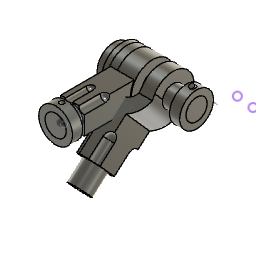
Knuckle Joint final_ (Autodesk Fusion 360 design; units mm, degrees)
Autodesk Fusion 360 part; units mm, degrees
sketch "Sketch1" plane through (0, 0, 0) normal (0, 1, 0) x (1, 0, 0) in component "eye"
  circle A0 centre (0, 0) radius 12.5
  dimension "d1" = 25
  constraint coincident A0.centre origin
  measures "d1" diameter of A0
extrude "Extrude1" add sketch "Sketch1" along normal blind 20 makes body 1 in component "eye"
sketch "Sketch2" plane through (0, 0, 0) normal (1, 0, 0) x (0, 1, 0) in component "eye"
sketch "Sketch3" plane through (0, 0, 0) normal (1, 0, 0) x (0, 1, 0) in component "eye"
  line L0 (20, 0) -> (100, 0)
  circle A0 centre (100, 0) radius 25
  circle A1 centre (100, 0) radius 12.5
  dimension "d4" = 80
  dimension "d5" = 50
  dimension "d6" = 25
  constraint coincident L0.end A0.centre
  constraint concentric A0 A1
  measures "d4" distance of L0.start L0.end
  measures "d5" diameter of A0
  measures "d6" diameter of A1
extrude "Extrude2" add sketch "Sketch3" along normal mid plane 30 separate body makes body 2 in component "eye"
sketch "Sketch4" plane through (0, 20, 0) normal (0, 1, 0) x (-1, 0, 0) in component "eye"
  circle A0 centre (0, 0) radius 12.5
sketch "Sketch1 (2)" plane through (0, 20, 0) normal (0, 1, 0) x (-1, 0, 0)
  line L0 (14, -14) -> (-14, -14)
  line L1 (-14, -14) -> (-14, 14)
  line L2 (-14, 14) -> (14, 14)
  line L3 (14, 14) -> (14, -14)
  line L4 (14, -14) -> (-14, 14) construction
  line L5 (-14, -14) -> (14, 14) construction
  dimension "d9" = 28
  dimension "d10" = 28
  constraint horizontal L0
  constraint perpendicular L0 L1
  constraint parallel L0 L2
  constraint parallel L1 L3
  constraint coincident L4 origin
  constraint coincident L5 origin
  measures "d9" distance of L0.start L0.end
  measures "d10" distance of L0.start L2.end
extrude "Extrude3" add sketch "Sketch1 (2)" along normal blind 60 bodies 1 2 in component "eye"
sketch "Sketch2 (2)" plane through (0, 0, 0) normal (0, 0, 1) x (1, 0, 0)
sketch "Sketch3 (2)" plane through (0, 0, 0) normal (0, 1, 0) x (1, 0, 0)
sketch "Sketch4 (2)" plane through (0, 0, 0) normal (0, 0, 1) x (1, 0, 0)
sketch "Sketch5" plane through (0, 0, 0) normal (0, 0, 1) x (1, 0, 0)
sketch "Sketch6" plane through (0, 0, 0) normal (0, 0, 1) x (1, 0, 0)
sketch "Sketch1 (3)" plane through (0, 0, 0) normal (0, 1, 0) x (1, 0, 0) in component "fork"
  arc A0 (3.8859, 308.1162) -> (3.8859, 278.1162) centre (3.8859, 293.1162) ccw
  arc A1 (3.8859, 323.1162) -> (3.8859, 263.1162) centre (3.8859, 293.1162) ccw
  line L0 (3.8859, 308.1162) -> (36.5811, 308.1162)
  line L1 (36.5811, 308.1162) -> (36.5811, 323.1162)
  line L2 (36.5811, 323.1162) -> (3.8859, 323.1162)
  line L3 (3.8859, 278.1162) -> (36.5811, 278.1162)
  line L4 (36.5811, 278.1162) -> (36.5811, 263.1162)
  line L5 (36.5811, 263.1162) -> (3.8859, 263.1162)
  line L6 (-22.6471, 307.1162) -> (-71.1141, 307.1162)
  line L7 (-71.1141, 307.1162) -> (-71.1141, 279.1162)
  line L8 (-71.1141, 279.1162) -> (-22.6471, 279.1162)
  dimension "d32" = 15
  dimension "d33" = 30
  dimension "d34" = 28
  dimension "d35" = 75
  constraint coincident A0.centre A1.centre
  constraint tangent A0 L0
  constraint horizontal L0
  constraint perpendicular L0 L1
  constraint tangent A1 L2
  constraint tangent A0 L3
  constraint parallel L2 L3
  constraint perpendicular L3 L4
  constraint tangent A1 L5
  constraint horizontal L6
  constraint perpendicular L6 L7
  constraint parallel L6 L8
  constraint coincident A1 L6.start
  constraint parallel L3 L5
  constraint parallel L0 L2
  constraint collinear L1 L4
  constraint coincident A1 L8.end
  constraint equal L6 L8
  measures "d32" radius of A0
  measures "d33" radius of A1
  measures "d34" distance of L6.end L7.end
  measures "d35" distance of A0.centre L7
extrude "Extrude1'" add sketch "Sketch1 (3)" along normal mid plane 56 separate body makes body 3 in component "fork"
sketch "Sketch2 (3)" plane through (0, 0, -263.1162) normal (0, 0, 1) x (-1, 0, 0) in component "fork"
  line L0 (-36.5811, 28) -> (-36.5811, -28)
  line L1 (-36.5811, -28) -> (-3.8859, -28)
  line L2 (-3.8859, -28) -> (-3.8859, 28)
  line L3 (-3.8859, 28) -> (-36.5811, 28)
  circle A0 centre (-11.5811, 0) radius 25
  circle A1 centre (-11.5811, 0) radius 12.5
  line L4 (1.9836, -21) -> (80, -21)
  line L5 (80, -21) -> (80, 21)
  line L6 (80, 21) -> (1.9836, 21)
  line L7 (1.9836, 21) -> (1.9836, -21)
  dimension "d38" = 50
  dimension "d39" = 25
  dimension "d40" = 42
  constraint concentric A0 A1
  constraint tangent L0 A0
  constraint horizontal L4
  constraint vertical L5
  constraint horizontal L6
  constraint vertical L7
  constraint coincident A0 L4.start
  constraint coincident A0 L6.end
  measures "d38" diameter of A0
  measures "d39" diameter of A1
  measures "d40" distance of L4.end L5.end
extrude "Extrude2'" cut sketch "Sketch2 (3)" against normal blind 80 contours L2 A0 A1 | L2 A0 A1 L7 | A0 L4 L5 L6 | A0 L7 keep common part bodies 3 in component "fork"
sketch "Sketch3 (3)" plane through (0, 0, 0) normal (0, 0, 1) x (1, 0, 0) in component "fork"
sketch "Sketch4 (3)" plane through (-71.1141, 0, 0) normal (-1, 0, 0) x (0, -1, 0) in component "fork"
  line L0 (21, -307.1162) -> (21, -279.1162)
  line L1 (21, -279.1162) -> (-21, -279.1162)
  line L2 (-21, -279.1162) -> (-21, -307.1162)
  line L3 (-21, -307.1162) -> (21, -307.1162)
  circle A0 centre (-0.0133, -293.1162) radius 12.5
  dimension "d45" = 25
  measures "d45" diameter of A0
extrude "Extrude3'" add sketch "Sketch4 (3)" along normal blind 25 contours A0 bodies 3 in component "fork"
sketch "Sketch5 (2)" plane through (0, 0, -279.1162) normal (0, 0, 1) x (-1, 0, 0) in component "fork"
  line L0 (71.1141, 21) -> (22.6471, 21)
  line L1 (22.6471, 21) -> (22.6471, -21)
  line L2 (22.6471, -21) -> (71.1141, -21)
  line L3 (71.1141, -21) -> (71.1141, 21)
  line L4 (71.1141, -12.4547) -> (48.3844, -12.4547)
  arc A0 (48.3844, -12.4547) -> (41.1141, -21) centre (48.3844, -19.82) ccw
  line L5 (71.1141, -21) -> (71.1141, -12.4547)
  dimension "d48" = 30
  dimension "d49" = 22.7298
  dimension "d50" = 7.3654
  constraint coincident L3 L4.start
  constraint perpendicular L3 L4
  constraint coincident L2 A0.end
  constraint tangent L4 A0
  constraint coincident L2.end L3.start
  measures "d48" horizontal distance of L4.start A0.end
  measures "d49" distance of L4.start L4.end
  measures "d50" radius of A0
revolve "Revolve1" cut sketch "Sketch5 (2)" angle 360 about axis through (-22.6471, 21, -279.1162) along (-1, 0, 0) contours L2 L3 L4 A0 L5 bodies 3 in component "fork"
sketch "Sketch6 (2)" plane through (0, 0, 0) normal (0, 0, 1) x (1, 0, 0) in component "fork"
sketch "Sketch7" plane through (0, 0, 0) normal (0, 0, 1) x (1, 0, 0) in component "fork"
sketch "Sketch7 (2)" plane through (0, 0, -79.4292) normal (0, 0, 1) x (-1, 0, 0)
  line L0 (128.0731, -132.4529) -> (150.8028, -132.4529)
  line L1 (150.8028, -132.4529) -> (150.8028, -98.9982)
  line L2 (150.8028, -98.9982) -> (102.3358, -98.9982)
  line L3 (102.3358, -98.9982) -> (102.3358, -140.9982)
  line L4 (102.3358, -140.9982) -> (120.8028, -140.9982)
  arc A0 (128.0731, -132.4529) -> (120.8028, -140.9982) centre (128.0731, -139.8183) ccw
  line L5 (150.8028, -107.545) -> (150.8028, -98.9982)
  line L6 (150.8028, -107.545) -> (128.0728, -107.545)
  arc A1 (120.8028, -98.9982) -> (128.0728, -107.545) centre (128.0728, -100.1796) ccw
  line L7 (150.8028, -98.9982) -> (120.8028, -98.9982)
  dimension "d52" = 22.73
  dimension "d53" = 30
  dimension "d54" = 7.3654
  constraint coincident L1 L5.start
  constraint coincident L1.end L2.start
  constraint perpendicular L2 L5
  constraint perpendicular L1 L6
  constraint coincident L2 A1.start
  constraint tangent L6 A1
  constraint equal A0 A1
  measures "d52" distance of L5.start L6.end
  measures "d53" horizontal distance of L5.start A1.start
  measures "d54" radius of A0
sketch "Sketch8" plane through (0, 0, -79.4292) normal (0, 0, 1) x (1, 0, 0)
sketch "Sketch9" plane through (0, 140.9982, 0) normal (0, 1, 0) x (-1, 0, 0)
  line L0 (150.8028, -87.9745) -> (128.0731, -87.9745)
  arc A0 (120.8028, -79.4292) -> (128.0731, -87.9745) centre (128.0731, -80.6092) ccw
  line L1 (120.8028, -79.4292) -> (102.3358, -79.4292)
  arc A1 (102.3358, -79.4292) -> (81.6723, -64.009) centre (75.8028, -93.4292) ccw
  line L2 (81.6723, -64.009) -> (81.6723, -79.6252)
  arc A2 (81.6723, -107.2332) -> (81.6723, -79.6252) centre (75.8028, -93.4292) ccw
  line L3 (81.6723, -107.2332) -> (81.6723, -122.8494)
  arc A3 (81.6723, -122.8494) -> (102.3358, -107.4292) centre (75.8028, -93.4292) ccw
  line L4 (102.3358, -107.4292) -> (150.8028, -107.4292)
  line L5 (150.8028, -107.4292) -> (150.8028, -87.9745)
  line L6 (150.8028, -107.4292) -> (150.8028, -98.8851)
  line L7 (150.8028, -98.8851) -> (128.0728, -98.8851)
  arc A4 (128.0728, -98.8851) -> (120.8028, -107.4292) centre (128.0728, -106.2501) ccw
  line L8 (120.8028, -107.4292) -> (150.8028, -107.4292)
  dimension "d58" = 30
  dimension "d59" = 7.365
  dimension "d60" = 22.73
  constraint coincident L4.end L5.start
  constraint coincident L5 L6.end
  constraint perpendicular L4 L6
  constraint perpendicular L5 L7
  constraint coincident L4 A4.end
  constraint tangent L7 A4
  measures "d58" horizontal distance of L6.end A4.end
  measures "d59" radius of A4
  measures "d60" distance of L6.end L7.end
sketch "Sketch10" plane through (0, 98.9982, 0) normal (0, -1, 0) x (1, 0, 0)
  arc A0 (-81.6723, -64.009) -> (-102.3358, -79.4292) centre (-75.8028, -93.4292) ccw
  line L0 (-102.3358, -79.4292) -> (-150.8028, -79.4292)
  line L1 (-150.8028, -79.4292) -> (-150.8028, -107.4292)
  line L2 (-150.8028, -107.4292) -> (-102.3358, -107.4292)
  arc A1 (-102.3358, -107.4292) -> (-81.6723, -122.8494) centre (-75.8028, -93.4292) ccw
  line L3 (-81.6723, -122.8494) -> (-81.6723, -107.2332)
  arc A2 (-81.6723, -79.6252) -> (-81.6723, -107.2332) centre (-75.8028, -93.4292) ccw
  line L4 (-81.6723, -79.6252) -> (-81.6723, -64.009)
revolve "Revolve2" cut sketch "Sketch7 (2)" angle 360 about axis through (-22.6471, -21, -279.1162) along (-1, 0, 0) contours L1 L2 L5 L6 A1 L7 sketch seen with x (1, 0, 0) y (0, 1, 0) z (0, 0, 1) at (79.6887, -119.9982, -199.687) bodies 3 in component "fork"
revolve "Revolve3" cut sketch "Sketch9" angle 360 about axis through (-22.6471, 21, -307.1162) along (-1, 0, 0) contours L4 L5 L6 L7 A4 L8 sketch seen with x (1, 0, 0) y (0, 1, 0) z (0, 0, 1) at (79.6887, -119.9982, -199.687) bodies 3 in component "fork"
sketch "Sketch11" plane through (0, 0, -107.4292) normal (0, 0, -1) x (1, 0, 0)
  arc A0 (-120.8028, -140.9982) -> (-128.0728, -132.4541) centre (-128.0728, -139.8191) ccw
  line L0 (-120.8028, -140.9982) -> (-102.3358, -140.9982)
  line L1 (-102.3358, -140.9982) -> (-102.3358, -98.9982)
  line L2 (-102.3358, -98.9982) -> (-150.8028, -98.9982)
  line L3 (-150.8028, -98.9982) -> (-150.8028, -132.4541)
  line L4 (-150.8028, -132.4541) -> (-128.0728, -132.4541)
  line L5 (-150.8028, -98.9982) -> (-150.8028, -107.0956)
  line L6 (-150.8028, -107.0956) -> (-128.0728, -107.0956)
  arc A1 (-128.0728, -107.0956) -> (-120.8028, -98.5514) centre (-128.0728, -99.7306) ccw
  line L7 (-120.8028, -98.5514) -> (-150.8028, -98.9982)
  dimension "d64" = 30
  dimension "d65" = 22.73
  dimension "d66" = 7.365
  constraint coincident L2.end L3.start
  constraint coincident L3 L5.end
  constraint perpendicular L2 L5
  constraint perpendicular L3 L6
  constraint tangent L6 A1
  constraint equal L4 L6
  constraint equal A0 A1
  measures "d64" horizontal distance of L5.end A1.end
  measures "d65" distance of L5.end L6.end
  measures "d66" radius of A1
revolve "Revolve4" cut sketch "Sketch11" angle 360 about axis through (-22.6471, -21, -307.1162) along (-1, 0, 0) contours L2 L3 L5 L6 A1 sketch seen with x (1, 0, 0) y (0, 1, 0) z (0, 0, 1) at (79.6887, -119.9982, -199.687) bodies 3 in component "fork"
sketch "Sketch1 (4)" plane through (0, 0, 0) normal (0, 1, 0) x (1, 0, 0) in component "pin"
  circle A0 centre (0, 0) radius 20
  dimension "d68" = 40
  constraint coincident A0.centre origin
  measures "d68" diameter of A0
extrude "Extrude1''" add sketch "Sketch1 (4)" along normal blind 12 separate body makes body 4 in component "pin"
sketch "Sketch2 (4)" plane through (0, 0, 0) normal (0, -1, 0) x (1, 0, 0) in component "pin"
  circle A0 centre (0, 0) radius 20
  circle A1 centre (0, 0) radius 12.5
  dimension "d71" = 25
  constraint coincident A0.centre A1.centre
  measures "d71" diameter of A1
extrude "Extrude2''" add sketch "Sketch2 (4)" along normal blind 86 contours A1 bodies 4 in component "pin"
sketch "Sketch3 (4)" plane through (0, 0, 0) normal (0, 0, 1) x (1, 0, 0) in component "pin"
sketch "Sketch4 (4)" plane through (0, 0, 0) normal (0, 1, 0) x (1, 0, 0) in component "pin"
sketch "Sketch1 (5)" plane through (0, 0, 0) normal (1, 0, 0) x (0, 0, -1) in component "collar"
  circle A0 centre (0, 0) radius 20
  circle A1 centre (0, 0) radius 12.5
  dimension "d74" = 40
  dimension "d75" = 25
  constraint coincident A0.centre A1.centre
  measures "d74" diameter of A0
  measures "d75" diameter of A1
extrude "Extrude1'''" add sketch "Sketch1 (5)" along normal blind 12 separate body makes body 5 in component "collar"
sketch "Sketch2 (5)" plane through (0, 0, 0) normal (0, 1, 0) x (1, 0, 0) in component "collar"
sketch "Sketch3 (5)" plane through (0, 0, 0) normal (0, 1, 0) x (1, 0, 0) in component "collar"
sketch "Sketch12" plane through (0, 0, 0) normal (1, 0, 0) x (0, 0, -1)
  circle A0 centre (0, -62.6322) radius 2
  line L0 (-10.0222, -74.6322) -> (14.9778, -74.6322)
  dimension "d80" = 4
  dimension "d81" = 12
  constraint vertical origin A0.centre
  measures "d80" diameter of A0
  measures "d81" distance of A0.centre L0
extrude "Extrude3''" cut sketch "Sketch12" along normal blind 28 sketch seen with x (1, 0, 0) y (0, 1, 0) z (0, 0, 1) at (-13.8456, -11.3678, 2.4778) bodies 4 in component "pin"
sketch "Sketch13" plane through (0, 0, 0) normal (0, 1, 0) x (1, 0, 0)
  circle A0 centre (0, 0) radius 20
  circle A1 centre (0, 0) radius 12.5
  dimension "d84" = 40
  dimension "d85" = 25
  constraint coincident A0.centre A1.centre
  constraint concentric A0 A1
  measures "d84" diameter of A0
  measures "d85" diameter of A1
extrude "Extrude1''''" add sketch "Sketch13" along normal blind 12 separate body makes body 6
sketch "Sketch14" plane through (0, 0, 0) normal (0, 0, 1) x (1, 0, 0)
  circle A0 centre (0, 7.0862) radius 2.75
  dimension "d88" = 5.5
  dimension "d89" = 5.5
  constraint vertical A0.centre origin
  measures "d88" diameter of A0
  measures "d89" diameter of A0
extrude "Extrude2'''" cut sketch "Sketch14" along normal mid plane 70 bodies 6
sketch "Sketch1 (6)" plane through (0, 0, 0) normal (1, 0, 0) x (0, 0, -1) in component "pin (1)"
ref_plane "WorkPlane1" through (0, 0, 50) normal (0, 0, 1) x (1, 0, 0) in component "pin (1)"
sketch "Sketch2 (6)" plane through (0, 0, 50) normal (0, 0, 1) x (1, 0, 0) in component "pin (1)"
ref_plane "WorkPlane2" through (50, 0, 0) normal (1, 0, 0) x (0, 1, 0) in component "pin (1)"
sketch "Sketch3 (6)" plane through (50, 0, 0) normal (1, 0, 0) x (0, 0, -1) in component "pin (1)"
  circle A0 centre (0, 0) radius 2.75
  dimension "d95" = 5.5
  constraint coincident A0.centre origin
  measures "d95" diameter of A0
loft "Loft1" add profiles "Sketch3 (6)" section 1 point at (0, 0, 0) section 2 separate body makes body 7 in component "pin (1)"
sketch "Sketch4 (5)" plane through (0, 0, 14) normal (0, 0, 1) x (-1, 0, 0) in component "pin (1)"
  line L0 (14, -20) -> (-14, -20)
sketch "Sketch5 (3)" plane through (0, 0, 14) normal (0, 0, 1) x (1, 0, 0) in component "eye"
  line L0 (-4.1354, 20) -> (0, 20)
  line L1 (0, 20) -> (0, 44.4385)
  arc A0 (0, 44.4385) -> (-4.1354, 50) centre (-5.8074, 44.4385) ccw
  line L2 (-4.1354, 50) -> (-4.1354, 20)
  point P0 (-15, 20)
  point P1 (0, 20)
  dimension "d97" = 30
  dimension "d98" = 5.8074
  dimension "d99" = 30
  dimension "d100" = 5.8074
  constraint horizontal L0
  constraint perpendicular L0 L1
  constraint tangent L1 A0
  constraint perpendicular L0 L2
  constraint coincident P1 L0.end
  measures "d97" vertical distance of A0.end P1
  measures "d98" radius of A0
  measures "d99" distance of L0.start A0.end
  measures "d100" radius of A0
revolve "Revolve1'" cut sketch "Sketch5 (3)" angle 360 about axis through (-4.1354, 50, 14) along (0, -1, 0) bodies 1 in component "eye"
sketch "Sketch6 (3)" plane through (0, 0, 14) normal (0, 0, 1) x (1, 0, 0) in component "eye"
  line L0 (7.5378, 19.887) -> (13.7926, 19.887)
  line L1 (7.5378, 19.887) -> (7.5378, 45.2451)
  arc A0 (13.7926, 49.887) -> (7.5378, 45.2451) centre (12.3876, 45.2451) ccw
  line L2 (13.7926, 49.887) -> (13.7926, 19.887)
  dimension "d102" = 30
  dimension "d103" = 25.3581
  dimension "d104" = 4.8498
  constraint horizontal L0
  constraint perpendicular L0 L1
  constraint tangent L1 A0
  constraint perpendicular L0 L2
  measures "d102" vertical distance of L0.start A0.start
  measures "d103" distance of L0.start L1.end
  measures "d104" radius of A0
revolve "Revolve2'" cut sketch "Sketch6 (3)" angle 360 about axis through (13.7926, 49.887, 14) along (0, -1, 0) bodies 1 in component "eye"
sketch "Sketch7 (3)" plane through (0, 0, -14) normal (0, 0, -1) x (1, 0, 0) in component "eye"
  line L0 (-14, -79.2877) -> (14, -79.2877)
  line L1 (14, -79.2877) -> (14, -20)
  line L2 (14, -20) -> (-14, -20)
  line L3 (-14, -20) -> (-14, -79.2877)
  line L4 (-14, -20) -> (-10, -20)
  constraint coincident L2.end L3.start
  constraint coincident L2 L4.end
  constraint perpendicular L3 L4
sketch "Sketch15" plane through (0, -85.0588, 0) normal (0, 1, 0) x (1, 0, 0)
  circle A0 centre (-74.0932, -8.4581) radius 2.75
  dimension "d106" = 5.5
  measures "d106" diameter of A0
extrude "Extrude2''''" cut sketch "Sketch15" along normal blind 30 sketch seen with x (1, 0, 0) y (0, 1, 0) z (0, 0, 1) at (79.5283, 85.0588, 5.5305) bodies 5 in component "collar"
component "eye" placed x (1, 0, 0) y (0, 1, 0) z (0, 0, 1) at (0, 0, 0)
component "fork" placed x (0, 0, 1) y (0, 1, 0) z (-1, 0, 0) at (-283.9098, 100, -11.5811)
component "pin" placed x (0, 1, 0) y (-1, 0, 0) z (0, 0, 1) at (-18.7886, 100, 0)
component "collar" placed x (-1, 0, 0) y (0, -1, 0) z (0, 0, 1) at (67.2114, 100, 0)
component "pin (1)" placed x (0, -1, 0) y (1, 0, 0) z (0, 0, 1) at (61.7763, 133.4544, 13.9886)
